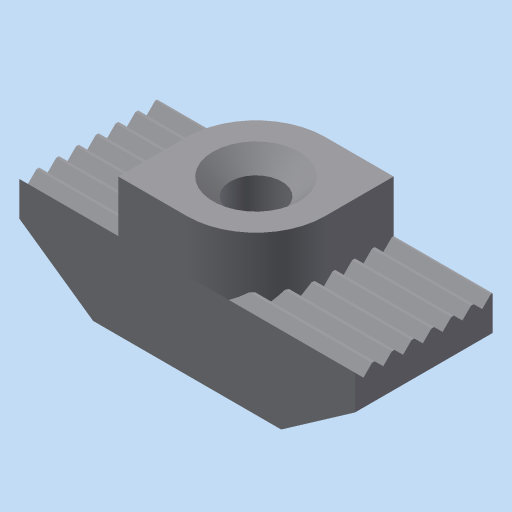
# Autodesk Inventor part: T-NUT - DropIn 4040 SERIES - M3
Saved by Autodesk Inventor 2023.2 (Build 272271000, 271)
## iProperties
Company: TraceParts S.A.
Created: 2023-02-26
Part Number: T-NUT - DropIn 4040 SERIES - M3
Checked By: TraceParts S.A.
Material: Generisch
Catalog Web Link: www.traceparts.com
Document SubType Name: Modeling
Designer: TraceParts
Density: 1 g/cm^3
Appearance: Vorgabe
REFERENCE: 07090-1008017
SUPPLIER: norelem
DESIGN: T-NUT FOR T-SLOT M08 STEEL
TraceParts.PartNumber: 30-06122017-106144
TraceParts.PartTitle: T-NUT FOR T-SLOT M08 STEEL
TraceParts.InstanceId: 30-06122017-1061443DYOD00EO1IYUO4TDSMY561GW
TRACEPARTS: TRACEPARTS
TraceParts.PartLanguage: en
TraceParts.PartVersion: 1.0.7
Author: TraceParts
Autodesk Inventor part; units mm, degrees
ref_plane "YZ Plane" through (0, 0, 0) normal (1, 0, 0) x (0, 1, 0)
ref_plane "XZ Plane" through (0, 0, 0) normal (0, 1, 0) x (-1, 0, 0)
ref_plane "XY Plane" through (0, 0, 0) normal (0, 0, 1) x (1, 0, 0)
sketch "Skizze3" plane through (0, 0, 0) normal (0, 0, 1) x (1, 0, 0)
  line L0 (0, 0) -> (5.4656, 0)
  line L1 (5.4656, 0) -> (9.75, 3)
  line L2 (9.75, 3) -> (9.75, 5)
  line L3 (9.75, 5) -> (0, 5)
  line L4 (0, 6) -> (0, -1) construction
  line L5 (0, 0) -> (-5.4656, 0)
  line L6 (-5.4656, 0) -> (-9.75, 3)
  line L7 (-9.75, 3) -> (-9.75, 5)
  line L8 (-9.75, 5) -> (0, 5)
  dimension "d6" = 9.75
  dimension "d8" = 5
  dimension "d9" = 3
  dimension "d10" = 145
  constraints: 16 end point, 3 symmetric about line, 2 perpendicular, 1 horizontal
  measures "d6" distance between parallel lines of L4 L2
  measures "d8" distance between parallel lines of L0 L3
  measures "d9" distance from line of L0 L1.end
  measures "d10" angle of L0 L1
extrude "Extrusion2" add sketch "Skizze3" along normal mid plane 8
sketch "Skizze4" plane through (-9.75, 5, 4) normal (0, 1, 0) x (1, 0, 0)
  line L0 (0, 8) -> (0, 0) projected
  line L1 (19.5, 0) -> (0, 0) projected
  line L2 (19.5, 8) -> (19.5, 0) projected
  line L3 (0, 8) -> (19.5, 8) projected
  circle A0 centre (9.75, 4) radius 1.5
  line L4 (5.75, 8) -> (13.75, 8)
  line L5 (13.75, 8) -> (13.75, 0)
  line L6 (13.75, 0) -> (5.75, 0)
  line L7 (5.75, 0) -> (5.75, 8)
  line L8 (5.75, 8) -> (13.75, 0) construction
  line L9 (13.75, 8) -> (5.75, 0) construction
  line L10 (0, 8) -> (19.5, 8) projected
  arc A1 (9.75, 8) -> (5.75, 4) centre (9.75, 4) ccw
  arc A2 (9.75, 0) -> (13.75, 4) centre (9.75, 4) ccw
  point P0 (9.75, 0)
  dimension "d13" = 3
  dimension "d14" = 8
  dimension "d15" = 8
  constraints: 12 end point, 4 midpoint, 4 point on circle, 3 centre point, 2 parallel, 2 symmetric about line, 1 coincident, 1 horizontal, 1 perpendicular, 1 other
  measures "d13" diameter of A0
  measures "d14" distance of L5.end L6.end
  measures "d15" distance of L4.end L5.end
extrude "Extrusion3" add sketch "Skizze4" along normal blind 3 and the other way blind 5 separate body contours L7 A1 L3 L5 A2 L1
sketch "Skizze5" plane through (9.75, 3, 4) normal (1, 0, 0) x (0, 0, -1)
  line L0 (8, 2) -> (0, 2) projected
  line L1 (0, 0) -> (0, 2) projected
  line L2 (8, 0) -> (0, 0) projected
  line L3 (8, 2) -> (8, 0) projected
  line L4 (0, 0) -> (0, 2) projected
  line L5 (0, 2) -> (0.495, 1.505)
  line L6 (0.495, 1.505) -> (0.9899, 2)
  line L7 (8, 2) -> (0, 2) projected
  line L8 (1.15, 2) -> (1.645, 1.505)
  line L9 (1.645, 1.505) -> (2.1399, 2)
  line L10 (2.3, 2) -> (2.795, 1.505)
  line L11 (2.795, 1.505) -> (3.2899, 2)
  line L12 (3.45, 2) -> (3.945, 1.505)
  line L13 (3.945, 1.505) -> (4.4399, 2)
  line L14 (4.6, 2) -> (5.095, 1.505)
  line L15 (5.095, 1.505) -> (5.5899, 2)
  line L16 (5.75, 2) -> (6.245, 1.505)
  line L17 (6.245, 1.505) -> (6.7399, 2)
  line L18 (6.9, 2) -> (7.395, 1.505)
  line L19 (7.395, 1.505) -> (7.8899, 2)
  point P0 (4, -3)
  dimension "d21" = 0.7
  dimension "d24" = 1.15
  constraints: 28 end point, 2 perpendicular, 1 horizontal, 1 point on line, 30 other
  measures "d21" distance of L0.end L5.end
  measures "d24" distance of L0.end L8.start
extrude "Extrusion4" cut sketch "Skizze5" against normal up to surface (19.5 mm away) contours L19 L18 L0 | L17 L16 L0 | L0 L6 L5 | L15 L14 L0 | L0 L9 L8 | L13 L12 L0 | L0 L11 L10 bodies 1
extrude "Extrusion5" cut sketch "Skizze4" against normal blind 10 contours A0 bodies 1
chamfer "Fase2" distance 1 angle 45 1 edges at (-1.5, 8, 0)
combine bodies "Kombinieren1" operation type add bodies to combine 2 1
